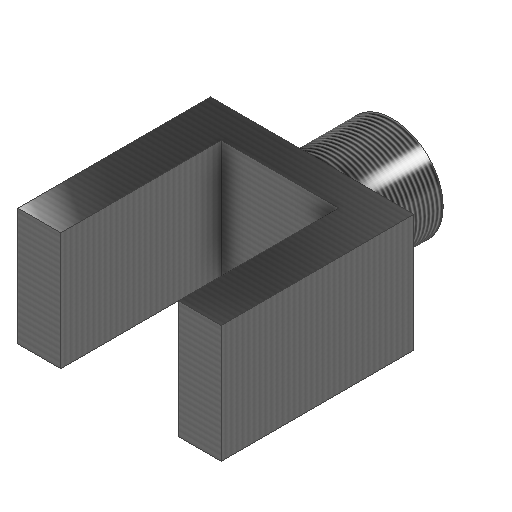
# Autodesk Inventor part: 08_Gripper
Saved by Autodesk Inventor 2022 (Build 260153000, 153)
## iProperties
Created: 2022-06-07
Part Number: 08_Gripper
Material: Generic
Document SubType Name: Sheet Metal
Designer: pzach
Density: 1 g/cm^3
Sheet Metal Rule: Default
Appearance: Engine Turned
Author: pzach
Autodesk Inventor part; units mm, degrees
ref_plane "YZ Plane" through (0, 0, 0) normal (1, 0, 0) x (0, 1, 0)
ref_plane "XZ Plane" through (0, 0, 0) normal (0, 1, 0) x (-1, 0, 0)
ref_plane "XY Plane" through (0, 0, 0) normal (0, 0, 1) x (1, 0, 0)
sketch "Sketch1" plane through (0, 0, 0) normal (0, 0, 1) x (1, 0, 0)
  line L0 (-190, 110) -> (-110, 110)
  line L1 (-110, 110) -> (-110, -110)
  line L2 (-110, -110) -> (-190, -110)
  line L3 (-190, -110) -> (-190, 110)
  line L4 (-190, 110) -> (-110, -110) construction
  line L5 (-110, 110) -> (-190, -110) construction
  line L6 (0, 0) -> (0, 2) construction
  line L7 (190, 110) -> (110, 110)
  line L8 (110, 110) -> (110, -110)
  line L9 (110, -110) -> (190, -110)
  line L10 (190, -110) -> (190, 110)
  line L11 (190, 110) -> (110, -110) construction
  line L12 (110, 110) -> (190, -110) construction
  point P0 (-150, 0)
  point P1 (-150, 0)
  point P2 (150, 0)
  point P3 (150, 0)
  dimension "d1" = 150
  dimension "d2" = 80
  dimension "d3" = 220
  dimension "d4" = 2
  constraints: 26 end point, 6 symmetric about line, 5 midpoint, 2 parallel, 1 horizontal, 1 horizontal alignment, 1 perpendicular, 1 vertical
  measures "d1" distance of L6.start point (-150, 0)
  measures "d2" distance of L0.start L0.end
  measures "d3" distance of L2.end L0.start
  measures "d4" distance of L6.start L6.end
extrude "Extrusion1" add sketch "Sketch1" against normal blind 300
sketch "Sketch2" plane through (0, 0, -300) normal (0, 0, -1) x (-1, 0, 0)
  line L0 (-110, 110) -> (-190, 110) projected
  line L1 (110, -110) -> (190, -110) projected
  line L2 (-190, 110) -> (190, 110)
  line L3 (190, 110) -> (190, -110)
  line L4 (190, -110) -> (-190, -110)
  line L5 (-190, -110) -> (-190, 110)
  point P0 (0, 0)
  constraints: 8 end point, 2 parallel, 1 horizontal, 1 perpendicular
extrude "Extrusion2" add sketch "Sketch2" along normal blind 60
sketch "Sketch3" plane through (0, 0, -360) normal (0, 0, -1) x (-1, 0, 0)
  circle A0 centre (0, 0) radius 95
  dimension "d9" = 190
  constraints: 2 coincident, 1 centre point
  measures "d9" diameter of A0
extrude "Extrusion3" add sketch "Sketch3" along normal blind 150
thread "Thread1" size "M190x8" class "6g" standard "ANSI Metric M Profile" full length
equation "\"BendRadius\" = Thickness"
equation "\"BendReliefWidth\" = Thickness"
equation "\"BendReliefDepth\" = 0.5 * Thickness"
equation "\"CornerReliefSize\" = 4 * Thickness"
equation "\"MinimumRemnant\" = 2 * Thickness"
equation "\"TransitionRadius\" = BendRadius"
equation "\"JacobiRadiusSize\" = BendRadius"
equation "\"GapSize\" = Thickness"
equation "\"Thickness\" = 3.048"
body "Solid1"
